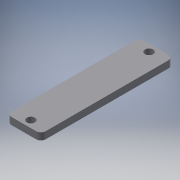
# Autodesk Inventor part: SteerServoClamp
Saved by Autodesk Inventor 2018 (Build 220112000, 112)
## iProperties
Created: 2018-05-19
Part Number: SteerServoClamp
Material: Generic
Document SubType Name: Modeling
Designer: reide
Density: 1 g/cm^3
Appearance: Default
Author: reide
Autodesk Inventor part; units mm, degrees
ref_plane "YZ Plane" through (0, 0, 0) normal (1, 0, 0) x (0, 1, 0)
ref_plane "XZ Plane" through (0, 0, 0) normal (0, 1, 0) x (-1, 0, 0)
ref_plane "XY Plane" through (0, 0, 0) normal (0, 0, 1) x (1, 0, 0)
sketch "Sketch1" plane through (0, 0, 0) normal (0, 0, 1) x (1, 0, 0)
  line L0 (9.9495, -14.97) -> (12.0175, -14.97) projected
  line L1 (9.9495, -20.042) -> (9.9495, -14.97) projected
  line L2 (4.9095, -20.042) -> (9.9495, -20.042) projected
  line L3 (4.9095, -15.47) -> (4.9095, -20.042) projected
  line L4 (-10.8425, -15.47) -> (4.9095, -15.47) projected
  line L5 (-10.8425, 10.39) -> (-10.8425, -15.47) projected
  line L6 (-7.5245, 10.39) -> (-10.8425, 10.39) projected
  line L7 (-7.5245, 30.75) -> (-7.5245, 10.39) projected
  line L8 (-12.0175, 30.75) -> (-7.5245, 30.75) projected
  line L9 (-12.0175, -25.67) -> (-12.0175, 30.75) projected
  line L10 (30.7975, -25.67) -> (-12.0175, -25.67) projected
  spline S0 degree 3 poles (31.7975, -27.4021) (31.7975, -27.1472) (31.7079, -26.8547) (31.4014, -26.2852) (31.0746, -25.9471) (30.7975, -25.67) knots 0.505532 0.505532 0.505532 0.505532 0.581995 0.581995 0.699558 0.699558 0.699558 0.699558 projected
  line L11 (31.7975, -32.02) -> (31.7975, -27.4021) projected
  line L12 (33.7975, -32.02) -> (31.7975, -32.02) projected
  line L13 (33.7975, -32.02) -> (33.7975, -17.51) projected
  line L14 (12.0175, -17.51) -> (33.7975, -17.51) projected
  line L15 (12.0175, -14.97) -> (12.0175, -17.51) projected
  line L16 (4.9095, 10.39) -> (-2.5085, 10.39) projected
  line L17 (4.9095, 14.962) -> (4.9095, 10.39) projected
  line L18 (9.9495, 14.962) -> (4.9095, 14.962) projected
  line L19 (9.9495, 9.89) -> (9.9495, 14.962) projected
  line L20 (12.0175, 9.89) -> (9.9495, 9.89) projected
  line L21 (12.0175, 22.59) -> (12.0175, 9.89) projected
  line L22 (33.7975, 22.59) -> (12.0175, 22.59) projected
  line L23 (33.7975, 22.59) -> (33.7975, 37.1) projected
  line L24 (31.7975, 37.1) -> (33.7975, 37.1) projected
  line L25 (31.7975, 32.4821) -> (31.7975, 37.1) projected
  spline S1 degree 3 poles (30.7975, 30.75) (31.0746, 31.0271) (31.4014, 31.3652) (31.7079, 31.9347) (31.7975, 32.2272) (31.7975, 32.4821) knots 0 0 0 0 0.117563 0.117563 0.194026 0.194026 0.194026 0.194026 projected
  line L26 (-2.5085, 30.75) -> (30.7975, 30.75) projected
  line L27 (-2.5085, 10.39) -> (-2.5085, 30.75) projected
  line L28 (10.0175, -25.67) -> (-0.5085, -25.67)
  line L29 (-2.5085, -23.67) -> (-2.5085, 28.75)
  line L30 (-0.5085, 30.75) -> (10.0175, 30.75)
  line L31 (12.0175, 28.75) -> (12.0175, -23.67)
  arc A0 (-2.5085, -23.67) -> (-0.5085, -25.67) centre (-0.5085, -23.67) ccw
  arc A1 (10.0175, -25.67) -> (12.0175, -23.67) centre (10.0175, -23.67) ccw
  arc A2 (-0.5085, 30.75) -> (-2.5085, 28.75) centre (-0.5085, 28.75) ccw
  arc A3 (12.0175, 28.75) -> (10.0175, 30.75) centre (10.0175, 28.75) ccw
  circle A4 centre (4.7545, -22.67) radius 1.625 projected
  circle A5 centre (4.7545, 27.75) radius 1.625 projected
  point P0 (0, 0)
  point P1 (12.0175, -25.67)
  dimension "d0" = 2
  constraints: 8 end point, 8 point on circle, 8 tangent, 5 point on line, 4 centre point, 3 equal radius, 2 parallel, 1 horizontal, 1 perpendicular
  measures "d0" radius of A0
extrude "Extrusion1" add sketch "Sketch1" along normal blind 3 contours L1 L2 L3 L4 L29 L16 L17 L18 L19 L20 L31 L0 | L0 L15 L31 A1 L10 A0 L29 L4 L3 L2 L1 | L20 L19 L18 L17 L16 L27 A2 L26 A3 L31 L21 | A4 | A5
sketch "Sketch2" plane through (0, 0, 3) normal (0, 0, 1) x (1, 0, 0)
  line L0 (9.9495, -14.97) -> (12.0175, -14.97) projected
  line L1 (9.9495, -20.042) -> (9.9495, -14.97) projected
  line L2 (4.9095, -20.042) -> (9.9495, -20.042) projected
  line L3 (4.9095, -15.47) -> (4.9095, -20.042) projected
  line L4 (-10.8425, -15.47) -> (4.9095, -15.47) projected
  line L5 (-10.8425, 10.39) -> (-10.8425, -15.47) projected
  line L6 (-7.5245, 10.39) -> (-10.8425, 10.39) projected
  line L7 (-7.5245, 30.75) -> (-7.5245, 10.39) projected
  line L8 (-12.0175, 30.75) -> (-7.5245, 30.75) projected
  line L9 (-12.0175, -25.67) -> (-12.0175, 30.75) projected
  line L10 (30.7975, -25.67) -> (-12.0175, -25.67) projected
  spline S0 degree 3 poles (31.7975, -27.4021) (31.7975, -27.1472) (31.7079, -26.8547) (31.4014, -26.2852) (31.0746, -25.9471) (30.7975, -25.67) knots 0.505532 0.505532 0.505532 0.505532 0.581995 0.581995 0.699558 0.699558 0.699558 0.699558 projected
  line L11 (31.7975, -32.02) -> (31.7975, -27.4021) projected
  line L12 (33.7975, -32.02) -> (31.7975, -32.02) projected
  line L13 (33.7975, -32.02) -> (33.7975, -17.51) projected
  line L14 (12.0175, -17.51) -> (33.7975, -17.51) projected
  line L15 (12.0175, -14.97) -> (12.0175, -17.51) projected
  line L16 (4.9095, 10.39) -> (-2.5085, 10.39) projected
  line L17 (4.9095, 14.962) -> (4.9095, 10.39) projected
  line L18 (9.9495, 14.962) -> (4.9095, 14.962) projected
  line L19 (9.9495, 9.89) -> (9.9495, 14.962) projected
  line L20 (12.0175, 9.89) -> (9.9495, 9.89) projected
  line L21 (12.0175, 22.59) -> (12.0175, 9.89) projected
  line L22 (33.7975, 22.59) -> (12.0175, 22.59) projected
  line L23 (33.7975, 22.59) -> (33.7975, 37.1) projected
  line L24 (31.7975, 37.1) -> (33.7975, 37.1) projected
  line L25 (31.7975, 32.4821) -> (31.7975, 37.1) projected
  spline S1 degree 3 poles (30.7975, 30.75) (31.0746, 31.0271) (31.4014, 31.3652) (31.7079, 31.9347) (31.7975, 32.2272) (31.7975, 32.4821) knots 0 0 0 0 0.117563 0.117563 0.194026 0.194026 0.194026 0.194026 projected
  line L26 (-2.5085, 30.75) -> (30.7975, 30.75) projected
  line L27 (-2.5085, 10.39) -> (-2.5085, 30.75) projected
  line L28 (-2.5085, 28.75) -> (-2.5085, -23.67) projected
  arc A0 (-2.5085, -23.67) -> (-0.5085, -25.67) centre (-0.5085, -23.67) ccw projected
  line L29 (-0.5085, -25.67) -> (10.0175, -25.67) projected
  arc A1 (10.0175, -25.67) -> (12.0175, -23.67) centre (10.0175, -23.67) ccw projected
  line L30 (12.0175, -23.67) -> (12.0175, 28.75) projected
  arc A2 (12.0175, 28.75) -> (10.0175, 30.75) centre (10.0175, 28.75) ccw projected
  line L31 (10.0175, 30.75) -> (-0.5085, 30.75) projected
  arc A3 (-0.5085, 30.75) -> (-2.5085, 28.75) centre (-0.5085, 28.75) ccw projected
  line L32 (-0.5085, -25.67) -> (10.0175, -25.67) projected
  line L33 (4.7545, -25.67) -> (4.7545, -22.67)
  circle A4 centre (4.7545, -22.67) radius 1.75
  line L34 (0, 0) -> (-38.7909, 0)
  line L35 (4.7545, 30.75) -> (4.7545, 27.75)
  circle A5 centre (4.7545, 27.75) radius 1.75
  circle A6 centre (4.7545, -22.67) radius 1.625 projected
  circle A7 centre (4.7545, 27.75) radius 1.625 projected
  dimension "d3" = 3
  dimension "d4" = 3.5
  dimension "d5" = 3
  dimension "d6" = 3.5
  constraints: 6 end point, 2 centre point, 2 coincident, 2 midpoint, 1 horizontal, 1 perpendicular, 1 vertical
  measures "d3" distance of L33.start L33.end
  measures "d4" diameter of A4
  measures "d5" distance of L35.start L35.end
  measures "d6" diameter of A5
extrude "Extrusion2" cut sketch "Sketch2" against normal blind 3 contours A6 | A4 | A7 | A5
body "Solid1"
